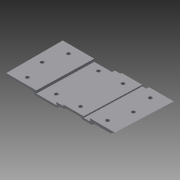
# Autodesk Inventor part: Finger_New_Support_base_Screwing
Saved by Autodesk Inventor 2015 (Build 190159000, 159)
## iProperties
Created: 2016-09-16
Part Number: Finger_New_Support_base_Screwing
Material: Generic
Document SubType Name: Modeling
Designer: Neelotpal Nag
Density: 1 g/cm^3
Appearance: Default
Author: Neelotpal Nag
Autodesk Inventor part; units mm, degrees
ref_plane "YZ Plane" through (0, 0, 0) normal (1, 0, 0) x (0, 1, 0)
ref_plane "XY Plane" through (0, 0, 0) normal (0, 0, 1) x (1, 0, 0)
sketch "Sketch1" plane through (0, 0, 0) normal (0, 0, 1) x (1, 0, 0)
  line L0 (0, 0) -> (81, 0)
  line L1 (0, 0) -> (0, -41.25)
  line L2 (0, -41.25) -> (76.5595, -41.25)
  line L3 (10.5, 0) -> (10.5, -41.25)
  line L4 (30.5, 0) -> (29.4198, -41.25)
  line L5 (30.5, 0) -> (71.7641, 0) construction
  line L6 (50.5, 0) -> (49.0595, -41.25)
  line L7 (70.5, 0) -> (68.699, -41.25)
  line L8 (78, 0) -> (76.5595, -41.25)
  line L9 (78, 0) -> (119.2751, 0) construction
  line L10 (76.5595, -41.25) -> (81, 0)
  line L11 (3, 0) -> (3, -41.25)
  line L12 (18, 0) -> (18, -41.25)
  line L13 (23, 0) -> (21.9198, -41.25)
  line L14 (23, 0) -> (64.2641, 0) construction
  line L15 (38, 0) -> (36.9198, -41.25)
  line L16 (38, 0) -> (79.2641, 0) construction
  line L17 (43, 0) -> (41.5595, -41.25)
  line L18 (43, 0) -> (84.2751, 0) construction
  line L19 (58, 0) -> (56.5595, -41.25)
  line L20 (58, 0) -> (99.2751, 0) construction
  line L21 (63, 0) -> (61.199, -41.25)
  line L22 (63, 0) -> (104.2893, 0) construction
  line L23 (29.4198, -41.25) -> (29.6031, -34.2524)
  line L24 (29.6031, -34.2524) -> (30.3884, -4.2627)
  line L25 (49.0595, -41.25) -> (49.234, -36.253)
  line L26 (49.234, -36.253) -> (50.281, -6.2713)
  line L27 (68.699, -41.25) -> (68.9171, -36.2548)
  line L28 (68.9171, -36.2548) -> (70.2257, -6.2833)
  circle A0 centre (10.5, -6.25) radius 1.25
  circle A1 centre (10.5, -36.25) radius 1.25
  circle A2 centre (30.3884, -4.2627) radius 1.25
  circle A3 centre (29.6031, -34.2524) radius 1.25
  circle A4 centre (50.281, -6.2713) radius 1.25
  circle A5 centre (49.234, -36.253) radius 1.25
  circle A6 centre (70.2257, -6.2833) radius 1.25
  circle A7 centre (68.9171, -36.2548) radius 1.25
  line L29 (10.5, -6.25) -> (10.5, -21.25)
  line L30 (10.5, -21.25) -> (6.218, -21.25)
  circle A8 centre (6.218, -21.25) radius 1.25
  line L31 (6.218, -21.25) -> (73.0178, -21.4249)
  line L32 (6.218, -21.25) -> (73.018, -21.25) construction
  circle A9 centre (73.0178, -21.4249) radius 1.25
  dimension "d10" = 92
  dimension "d11" = 91.5
  dimension "d12" = 91.5
  dimension "d13" = 92
  dimension "d14" = 92
  dimension "d15" = 92.5
  dimension "d67" = 2.5
  dimension "d68" = 2.5
  dimension "d69" = 2.5
  dimension "d70" = 2.5
  dimension "d71" = 2.5
  dimension "d72" = 2.5
  dimension "d73" = 2.5
  dimension "d74" = 2.5
  dimension "d77" = 15
  dimension "d78" = 4.282
  dimension "d79" = 2.5
  dimension "d80" = 66.8
  dimension "d81" = 0.15
  dimension "d82" = 2.5
  constraints: 62 end point, 19 coincident, 10 centre point, 9 horizontal, 9 point on line, 8 equal length, 5 vertical, 29 other
  measures "d10" angle of L8 L9
  measures "d11" angle of L13 L14
  measures "d12" angle of L15 L16
  measures "d13" angle of L17 L18
  measures "d14" angle of L19 L20
  measures "d15" angle of L21 L22
  measures "d67" diameter of A0
  measures "d68" diameter of A1
  measures "d69" diameter of A2
  measures "d70" diameter of A3
  measures "d71" diameter of A4
  measures "d72" diameter of A5
  measures "d73" diameter of A6
  measures "d74" diameter of A7
  measures "d77" distance of L29.start L29.end
  measures "d78" distance of L29.end L30.end
  measures "d79" diameter of A8
  measures "d80" distance of L31.start L31.end
  measures "d81" angle of L31 L32
  measures "d82" diameter of A9
sketch "Sketch2" plane through (0, 0, 0) normal (0, 1, 0) x (-1, 0, 0)
  line L0 (-43, 0) -> (-58, 0)
  line L1 (-58, 0) -> (-58, 1)
  line L2 (-58, 1) -> (-43, 1)
  line L3 (-43, 1) -> (-43, 0)
  line L4 (-64.4672, 0) -> (-78, 0)
  line L5 (-78, 0) -> (-78, 2)
  line L6 (-78, 2) -> (-63, 2)
  line L7 (-63, 2) -> (-63, 0)
  line L8 (-23, 0) -> (-21.9198, 0) projected
  line L9 (-30.5, 0) -> (-29.4198, 0) projected
  line L10 (-23, 0) -> (-38, 0)
  line L11 (-38, 0) -> (-38, -2)
  line L12 (-38, -2) -> (-23, -2)
  line L13 (-23, -2) -> (-23, 0)
  line L14 (0, 0) -> (-23, 0)
  line L15 (-23, 0) -> (-23, -1.5)
  line L16 (-21.5, -1.5) -> (0, -1.5)
  line L17 (0, -1.5) -> (0, 0)
  line L18 (-23, 0) -> (-21.5, 0)
  line L19 (-21.5, -1.5) -> (-21.5, -3.5)
  line L20 (-21.5, -3.5) -> (-23, -3.5)
  line L21 (-23, -2) -> (-23, 0)
  line L22 (-23, -2) -> (-38, -2)
  line L23 (-39.5, -2) -> (-39.5, -3.5)
  line L24 (-39.5, -3.5) -> (-23, -3.5)
  line L25 (-39.5, -2) -> (-39.5, -1.5)
  line L26 (-39.5, 0) -> (-38, 0)
  line L27 (-38, 0) -> (-38, -2)
  line L28 (-38, 0) -> (-43, 0)
  line L29 (-43, -0.5) -> (-43, -1.5)
  line L30 (-43, -1.5) -> (-39.5, -1.5)
  line L31 (-38, -1.5) -> (-38, 0)
  line L32 (-43, 1) -> (-58, 1)
  line L33 (-58, 1) -> (-58, 0)
  line L34 (-56.5, -0.5) -> (-44, -0.5)
  line L35 (-43, -0.5) -> (-43, 1)
  line L36 (-38, 0) -> (-44, 0)
  line L37 (-44, -0.5) -> (-44, -1.5)
  line L38 (-44, -1.5) -> (-38, -1.5)
  line L39 (-38, -1.5) -> (-38, 0)
  line L40 (-56.5, 0) -> (-63, 0)
  line L41 (-64.4672, 0) -> (-64.4672, -1.5)
  line L42 (-64.4672, -1.5) -> (-56.5, -1.5)
  line L43 (-56.5, -1.5) -> (-56.5, -0.5)
  line L44 (-81, 2) -> (-78, 2)
  line L45 (-81, 2) -> (-78, 0)
  line L46 (-18, 0) -> (-18, -1.5)
  line L47 (0, 0) -> (-18, 0)
  line L48 (-18, 0) -> (-18, -1.5)
  line L49 (-18, -1.5) -> (0, -1.5)
  line L50 (0, -1.5) -> (0, 0)
  line L51 (-18, -1.5) -> (-18, 0)
  line L52 (-23, 0) -> (-23, -2)
  line L53 (-38, -2) -> (-38, 0)
  line L54 (-43, 0) -> (-43, -1.5)
  line L55 (-18, -1.5) -> (-21.5, -1.5)
  line L56 (-38, -2) -> (-23, -2)
  line L57 (-23, -2) -> (-23, 0)
  line L58 (-23, 0) -> (-18, 0)
  line L59 (-18, 0) -> (-18, -1.5)
  line L60 (-18, 0) -> (-23, 0)
  line L61 (-23, 0) -> (-23, -1.5)
  line L62 (-23, -1.5) -> (-18, -1.5)
  line L63 (-18, -1.5) -> (-18, 0)
  line L64 (-23, 0) -> (-21.5, 0)
  line L65 (-21.5, 0) -> (-21.5, -3.5)
  line L66 (-21.5, -3.5) -> (-23, -3.5)
  line L67 (-23, -3.5) -> (-23, 0)
  line L68 (-21.5, -3.5) -> (-39.5, -3.5)
  line L69 (-39.5, -3.5) -> (-39.5, -2)
  line L70 (-39.5, -2) -> (-21.5, -2)
  line L71 (-21.5, -2) -> (-21.5, -3.5)
  line L72 (-39.5, -2) -> (-38, -2)
  line L73 (-38, -2) -> (-38, 0)
  line L74 (-38, 0) -> (-39.5, 0)
  line L75 (-39.5, 0) -> (-39.5, -2)
  line L76 (-38, 0) -> (-44, 0)
  line L77 (-44, 0) -> (-44, -1.5)
  line L78 (-44, -1.5) -> (-38, -1.5)
  line L79 (-38, -1.5) -> (-38, 0)
  line L80 (-44, -0.5) -> (-58, -0.5)
  line L81 (-58, -0.5) -> (-58, 1)
  line L82 (-58, 1) -> (-44, 1)
  line L83 (-44, 1) -> (-44, -0.5)
  line L84 (-58, 1) -> (-56.5, 1)
  line L85 (-56.5, 1) -> (-56.5, -1.5)
  line L86 (-56.5, -1.5) -> (-58, -1.5)
  line L87 (-58, -1.5) -> (-58, 1)
  line L88 (-56.5, -1.5) -> (-64.4672, -1.5)
  line L89 (-64.4672, -1.5) -> (-64.4672, 0)
  line L90 (-64.4672, 0) -> (-56.5, 0)
  line L91 (-56.5, 0) -> (-56.5, -1.5)
  line L92 (-63, 0) -> (-78, 0)
  line L93 (-78, 0) -> (-78, 2)
  line L94 (-78, 2) -> (-63, 2)
  line L95 (-63, 2) -> (-63, 0)
  point P0 (-50.5, 0)
  point P1 (-58, 0)
  point P2 (-70.5, 0)
  point P3 (-81, 0)
  dimension "d24" = 1.5
  dimension "d29" = 6
  constraints: 188 end point, 43 parallel, 24 perpendicular, 20 horizontal, 7 point on line, 3 collinear
  measures "d24" distance of L15.end L14.end
  measures "d29" distance of L38.end L37.end
ref_plane "Work Plane1" through (0, -41.25, 0) normal (0, 1, 0) x (-1, 0, 0)
sketch "Sketch3" plane through (0, -41.25, 0) normal (0, 1, 0) x (-1, 0, 0)
  line L0 (-23, 0) -> (-21.9198, 0) projected
  line L1 (-30.5, 0) -> (-29.4198, 0) projected
  line L2 (-38, 0) -> (-36.9198, 0) projected
  line L3 (-43, 0) -> (-41.5595, 0) projected
  line L4 (-50.5, 0) -> (-49.0595, 0) projected
  line L5 (-58, 0) -> (-56.5595, 0) projected
  line L6 (-63, 0) -> (-61.199, 0) projected
  line L7 (-70.5, 0) -> (-68.699, 0) projected
  line L8 (-78, 0) -> (-76.5595, 0) projected
  point P0 (0, 0)
  point P1 (-3, 0)
  point P2 (-3, 0)
  point P3 (-3, 0)
  point P4 (-10.5, 0)
  point P5 (-10.5, 0)
  point P6 (-10.5, 0)
  point P7 (-18, 0)
  point P8 (-18, 0)
  point P9 (-18, 0)
sketch "Sketch4" plane through (0, -41.25, 0) normal (0, 1, 0) x (-1, 0, 0)
  line L0 (0, 0) -> (-76.5595, 0) projected
  line L1 (-23, 0) -> (-21.9198, 0) projected
  line L2 (-30.5, 0) -> (-29.4198, 0) projected
  line L3 (-38, 0) -> (-36.9198, 0) projected
  line L4 (-43, 0) -> (-41.5595, 0) projected
  line L5 (-50.5, 0) -> (-49.0595, 0) projected
  line L6 (-58, 0) -> (-56.5595, 0) projected
  line L7 (-63, 0) -> (-61.199, 0) projected
  line L8 (-70.5, 0) -> (-68.699, 0) projected
  line L9 (-78, 0) -> (-76.5595, 0) projected
  line L10 (-21.9198, 0) -> (-36.9198, 0)
  line L11 (-36.9198, 0) -> (-36.9198, -2)
  line L12 (-36.9198, -2) -> (-21.9198, -2)
  line L13 (-21.9198, -2) -> (-21.9198, 0)
  line L14 (-41.5595, 0) -> (-56.5595, 0)
  line L15 (-56.5595, 0) -> (-56.5595, 1)
  line L16 (-56.5595, 1) -> (-41.5595, 1)
  line L17 (-41.5595, 1) -> (-41.5595, 0)
  line L18 (-61.199, 0) -> (-76.199, 0)
  line L19 (-76.199, 0) -> (-76.199, 2)
  line L20 (-76.199, 2) -> (-61.199, 2)
  line L21 (-61.199, 2) -> (-61.199, 0)
  point P0 (-3, 0)
  point P1 (-3, 0)
  point P2 (-3, 0)
  point P3 (-10.5, 0)
  point P4 (-10.5, 0)
  point P5 (-10.5, 0)
  point P6 (-18, 0)
  point P7 (-18, 0)
  point P8 (-18, 0)
  point P9 (-3, 0)
  point P10 (-10.5, 0)
  point P11 (-18, 0)
  dimension "d17" = 15
  dimension "d18" = 2
  dimension "d19" = 1
  dimension "d20" = 15
  dimension "d21" = 2
  constraints: 24 end point, 12 coincident, 6 parallel, 3 horizontal, 3 perpendicular, 1 other
  measures "d17" distance of L12.end L11.end
  measures "d18" distance of L11.end L10.end
  measures "d19" distance of L14.end L15.end
  measures "d20" distance of L19.end L20.end
  measures "d21" distance of L18.end L19.end
sketch "Sketch5" plane through (0, 0, 0) normal (0, 1, 0) x (-1, 0, 0)
  point P0 (0, 0)
sweep "Sweep1" add profiles "Sketch2" path "Sketch1" path curves L3 contours L14 L17 L16 L46
sweep "Sweep2" add profiles "Sketch2" path "Sketch1" path curves L13 contours L8 L14 L65 L62 L13 | L14 L46 L16 L65
sweep "Sweep3" add profiles "Sketch2" path "Sketch1" path curves L4 contours L70 L12 L67 L24 L23 | L70 L19 L20 L67
sweep "Sweep4" add profiles "Sketch2" path "Sketch1" path curves L4 contours L70 L19 L20 L67 | L13 L62 L19 L70
sketch3d "3D Sketch1"
  line L0 (39.5, 0, -2) -> (38.4198, -41.25, -2)
sweep "Sweep5" add profiles "Sketch2" path "3D Sketch1" contours L26 L11 L38 L75 | L38 L11 L70 L25
sweep "Sweep6" add profiles "Sketch2" path "Sketch1" path curves L17 contours L35 L29 L38 L37 L77 L0 | L28 L75 L30 L29 L35 | L26 L11 L38 L75
sweep "Sweep7" add profiles "Sketch2" path "Sketch1" path curves L6 contours L0 L83 L2 L3 | L0 L85 L2 L83 | L0 L1 L2 L85
sweep "Sweep8" add profiles "Sketch2" path "Sketch1" path curves L6 contours L77 L34 L85 L0 | L0 L85 L2 L83 | L85 L80 L81 L0 | L0 L1 L2 L85
sweep "Sweep9" add profiles "Sketch2" path "Sketch1" path curves L19 contours L85 L80 L81 L0 | L0 L1 L2 L85 | L43 L42 L87 L80
sketch3d "3D Sketch2"
  line L0 (58, 0, 1) -> (56.5595, -41.25, 1)
sweep "Sweep10" add profiles "Sketch2" path "3D Sketch2" contours L85 L80 L81 L0 | L81 L87 L42 L41 L90 L40 | L43 L42 L87 L80
sweep "Sweep11" add profiles "Sketch2" path "Sketch1" path curves L21 contours L90 L4 L5 L6 L7
sketch3d "3D Sketch3"
  line L0 (78, 0, 2) -> (76.199, -41.25, 2)
sweep "Sweep12" add profiles "Sketch2" path "3D Sketch3" contours L5 L45 L44
fillet "Fillet1" radius 2 1 edges at (77.0995, -20.625, 0)
fillet "Fillet2" radius 2 2 edges at (63.7469, -20.625, -1.5) (63.7469, -20.625, 0)
fillet "Fillet3" radius 1 2 edges at (55.7798, -20.625, -1.5) (55.7798, -20.625, -0.5)
fillet "Fillet4" radius 2 2 edges at (43.2798, -20.625, -0.5) (43.2798, -20.625, -1.5)
fillet "Fillet5" radius 2 2 edges at (38.9599, -20.625, -1.5) (38.9599, -20.625, -3.5)
fillet "Fillet6" radius 2 2 edges at (20.9599, -20.625, -3.5) (20.9599, -20.625, -1.5)
fillet "Fillet7" radius 2 1 edges at (0, -20.625, -1.5)
extrude "Extrusion1" cut sketch "Sketch1" along normal through all both and the other way through all contours A0 L3 | L3 A0 | A1 L3 | L3 A1 | A2 L4 | L4 A2 | A3 L4 | L4 A3 | A4 L6 | L6 A4 | A5 L6 | L6 A5 | A6 L7 | L7 A6 | A7 L7 | L7 A7
extrude "Extrusion2" cut sketch "Sketch1" along normal through all both and the other way through all contours L31 L30 A8 | A8 L30 L31 | A9
body "Solid1"
